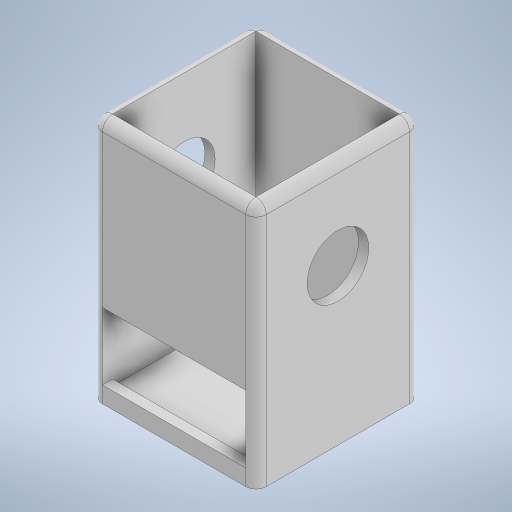
# Autodesk Inventor part: Dispenser
Saved by Autodesk Inventor 2024.2 (Build 282272000, 272)
## iProperties
Created: 2024-02-24
Part Number: Dispenser
Material: Generic
Document SubType Name: Modeling
Designer: Luke
Density: 1 g/cm^3
Appearance: Default
Author: Luke
Autodesk Inventor part; units mm, degrees
ref_plane "YZ Plane" through (0, 0, 0) normal (1, 0, 0) x (0, 1, 0)
ref_plane "XZ Plane" through (0, 0, 0) normal (0, 1, 0) x (-1, 0, 0)
ref_plane "XY Plane" through (0, 0, 0) normal (0, 0, 1) x (1, 0, 0)
sketch "Sketch1" plane through (0, 0, 0) normal (0, 1, 0) x (-1, 0, 0)
  line L0 (0, 0) -> (-50.8, 0)
  line L1 (-50.8, 0) -> (-50.8, 50.8)
  line L2 (-50.8, 50.8) -> (0, 50.8)
  line L3 (0, 50.8) -> (0, 0)
  dimension "d0" = 50.8
  dimension "d1" = 50.8
  constraints: 8 end point, 2 parallel, 1 horizontal, 1 perpendicular
  measures "d0" distance of L1.end L2.end
  measures "d1" distance between parallel lines of L0 L2
extrude "Extrusion1" add sketch "Sketch1" along normal blind 3.175
sketch "Sketch2" plane through (0, 3.175, 0) normal (0, 1, 0) x (1, 0, 0)
  line L0 (3.175, -47.625) -> (47.625, -47.625)
  line L1 (47.625, -47.625) -> (47.625, -3.175)
  line L2 (47.625, -3.175) -> (3.175, -3.175)
  line L3 (3.175, -3.175) -> (3.175, -47.625)
  line L4 (50.8, 0) -> (0, 0) projected
  line L5 (0, 0) -> (0, -50.8) projected
  line L6 (0, -50.8) -> (50.8, -50.8) projected
  line L7 (50.8, -50.8) -> (50.8, 0) projected
  dimension "d4" = 3.175
  dimension "d5" = 3.175
  dimension "d6" = 3.175
  dimension "d7" = 3.175
  constraints: 8 end point, 2 parallel, 1 horizontal, 1 perpendicular
  measures "d4" distance between parallel lines of L4 L2
  measures "d5" distance between parallel lines of L5 L3
  measures "d6" distance between parallel lines of L6 L0
  measures "d7" distance between parallel lines of L7 L1
extrude "Extrusion2" add sketch "Sketch2" along normal blind 73.025
sketch "Sketch3" plane through (0, 0, 50.8) normal (0, 0, 1) x (1, 0, 0)
  line L0 (3.175, 25.8698) -> (47.625, 25.8698)
  line L1 (47.625, 25.8698) -> (47.625, 5.08)
  line L2 (47.625, 5.08) -> (3.175, 5.08)
  line L3 (3.175, 5.08) -> (3.175, 25.8698)
  line L4 (3.175, 3.175) -> (47.625, 3.175) projected
  line L5 (0, 0) -> (50.8, 0) projected
  line L6 (0, 0) -> (0, 76.2) projected
  line L7 (50.8, 0) -> (50.8, 76.2) projected
  dimension "d11" = 5.08
  dimension "d12" = 3.175
  dimension "d13" = 3.175
  constraints: 8 end point, 2 parallel, 1 horizontal, 1 perpendicular
  measures "d11" distance between parallel lines of L2 L5
  measures "d12" distance between parallel lines of L6 L3
  measures "d13" distance between parallel lines of L7 L1
extrude "Extrusion3" cut sketch "Sketch3" against normal blind 3.175
sketch "Sketch6" plane through (50.8, 0, 50.8) normal (1, 0, 0) x (0, 0, -1)
  line L0 (0, 0) -> (0, 76.2) projected
  line L1 (0, 88.8381) -> (50.8, 88.8381)
  line L2 (50.8, 0) -> (50.8, 76.2) projected
  circle A0 centre (25.4, 48.1981) radius 9.525
  dimension "d16" = 19.05
  dimension "d17" = 40.64
  constraints: 2 end point, 2 point on line, 1 centre point, 1 horizontal
  measures "d16" diameter of A0
  measures "d17" distance from line of L1 A0.centre
extrude "Extrusion4" cut sketch "Sketch6" against normal blind 50.8
fillet "Fillet1" radius 3.175 4 edges at (0, 38.1, 50.8) (0, 38.1, 0) (50.8, 38.1, 50.8) (50.8, 38.1, 0)
fillet "Fillet2" radius 3.175 8 edges at (0.9299, 76.2, 49.8701) (25.4, 76.2, 50.8) (49.8701, 76.2, 49.8701) (50.8, 76.2, 25.4) (49.8701, 76.2, 0.9299) (25.4, 76.2, 0) (0.9299, 76.2, 0.9299) (0, 76.2, 25.4)
body "Solid1"
